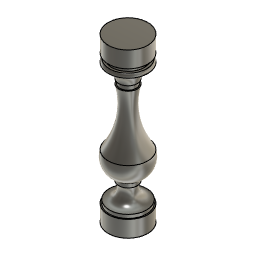
Sketch25_Final v2 (Autodesk Fusion 360 design; units mm, degrees)
Autodesk Fusion 360 part; units mm, degrees
sketch "Sketch1" plane through (0, 0, 0) normal (0, 1, 0) x (1, 0, 0)
  line L0 (0, 0) -> (8.5, 0)
  line L1 (0, 0) -> (0, -70)
  line L2 (8.5, 0) -> (8.5, -7)
  line L3 (8.5, -7) -> (8, -7)
  line L4 (8, -7) -> (8, -8.5)
  line L5 (8.5, -7) -> (0, -7)
  line L6 (8, -8.5) -> (0, -8.5)
  line L7 (0, -8.5) -> (0, -15.5)
  line L8 (0, -15.5) -> (4, -15.5)
  arc A0 (8, -8.5) -> (4, -15.5) centre (8, -13.1429) ccw
  line L9 (4, -15.5) -> (4, -17.5)
  line L10 (4, -17.5) -> (0, -17.5)
  line L11 (0, -17.5) -> (4.5, -17.5)
  line L12 (0, -17.5) -> (0, -27)
  line L13 (0, -27) -> (8.5, -27)
  arc A1 (8.5, -27) -> (4.5, -17.5) centre (0.9117, -24.603) ccw
  line L14 (0, -27) -> (0, -51.5)
  line L15 (0, -51.5) -> (4, -51.5)
  arc A2 (8.5, -27) -> (4, -51.5) centre (33.8925, -44.3272) ccw
  line L16 (0, -51.5) -> (3.5, -51.5)
  line L17 (3.5, -51.5) -> (3.5, -53.5)
  line L18 (3.5, -53.5) -> (0, -53.5)
  line L19 (0, -53.5) -> (4, -53.5)
  line L20 (0, -53.5) -> (0, -59.5)
  line L21 (0, -59.5) -> (8.5, -59.5)
  arc A3 (4, -53.5) -> (8.5, -59.5) centre (10.7181, -53.1489) ccw
  line L22 (0, -59.5) -> (0, -61)
  line L23 (0, -61) -> (8, -61)
  line L24 (0, -61) -> (7, -61)
  line L25 (7, -61) -> (7, -63)
  line L26 (7, -63) -> (0, -63)
  line L27 (0, -63) -> (8.5, -63)
  line L28 (8.5, -63) -> (8.5, -70)
  line L29 (8.5, -70) -> (0, -70)
  arc A4 (8, -61) -> (8.5, -59.5) centre (7.0099, -59.8366) ccw
  dimension "d2" = 70
  dimension "d3" = 7
  dimension "d5" = 1.5
  dimension "d7" = 7
  dimension "d12" = 2
  dimension "d15" = 9.5
  dimension "d17" = 24.5
  dimension "d20" = 2
  dimension "d22" = 6
  dimension "d24" = 1.5
  dimension "d26" = 2
  dimension "d29" = 7
  constraint coincident L0.start L1.start
  constraint coincident L1 L5.end
  constraint coincident L1 L6.end
  constraint coincident L1 L18.end
  measures "d2" distance of L0.start L1.end
  measures "d3" distance of L0.end L2.end
  measures "d5" distance of L3.end L4.end
  measures "d7" distance of L6.end L7.end
  measures "d12" distance of L8.end L9.end
  measures "d15" distance of L10.end L12.end
  measures "d17" distance of L12.end L14.end
  measures "d20" distance of L16.end L17.end
  measures "d22" distance of L18.end L20.end
  measures "d24" distance of L20.end L22.end
  measures "d26" distance of L24.end L25.end
  measures "d29" distance of L27.end L28.end
revolve "Revolve1" add sketch "Sketch1" angle 360 about axis through (0, 0, 0) along (0, 0, 1)
